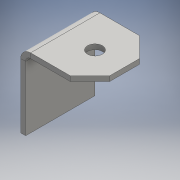
# Autodesk Inventor part: Part120
Saved by Autodesk Inventor 2016 (Build 200138000, 138)
## iProperties
Created: 2018-11-16
Part Number: Part120
Material: Generic
Document SubType Name: Sheet Metal
Designer: hovm
Density: 1 g/cm^3
Sheet Metal Rule: Default_mm
Appearance: Default
Author: hovm
Autodesk Inventor part; units mm, degrees
ref_plane "YZ Plane" through (0, 0, 0) normal (1, 0, 0) x (0, 1, 0)
ref_plane "XZ Plane" through (0, 0, 0) normal (0, 1, 0) x (-1, 0, 0)
ref_plane "XY Plane" through (0, 0, 0) normal (0, 0, 1) x (1, 0, 0)
sketch "Sketch1" plane through (0, 0, 0) normal (0, 0, 1) x (1, 0, 0)
  line L0 (-7, -7) -> (7, -7)
  line L1 (7, -7) -> (7, 7)
  line L2 (7, 7) -> (-7, 7)
  line L3 (-7, 7) -> (-7, -7)
  line L4 (-7, -7) -> (7, 7) construction
  line L5 (7, -7) -> (-7, 7) construction
  point P0 (0, 0)
  dimension "d0" = 14
  dimension "d1" = 14
  measures "d0" distance of L1.end L2.end
  measures "d1" distance of L0.end L1.end
extrude "Plate1" add sketch "Sketch1" along normal blind 1
sketch "Sketch2" plane through (-6, 7, 1) normal (-1, 0, 0) x (0, -1, 0)
  line L0 (14, 0) -> (0, 0)
  line L1 (0, 0) -> (0, -15)
  line L2 (0, -15) -> (14, -15)
  line L3 (14, -15) -> (14, 0)
  constraints: 6 end point, 1 horizontal, 1 perpendicular, 1 vertical
edge flange "Flange1" height 15 angle 90 thickness 1 bend radius 1 thickness toward (-1, 0, 0) relief tear relief width 1 relief depth 0.5 edges at (-7, 0, 0) wall of the first edge with corners at (-6, -7, 1) (-6, 7, 1) (-6, 7, -14) (-6, -7, -14)
bend "Bend1"
corner "Corner1"
sketch "Sketch3" plane through (0, 0, 1) normal (0, 0, 1) x (1, 0, 0)
  line L0 (7, -7) -> (7, 7) projected
  point P0 (0, 0)
  point P1 (1, 0)
  point P2 (7, 0)
  dimension "d13" = 6
  constraints: 1 horizontal alignment, 1 midpoint
  measures "d13" distance from line of L0 point (1, 0)
hole "Hole1" at (1, 0, 1) direction (0, 0, -1) diameter 3 depth 1 tip angle 118
chamfer "Corner Chamfer1" distance 4 angle 45 2 edges at (7, 7, 0.5) (7, -7, 0.5)
equation "\"d1\" = d0"
equation "\"d19\" = Thickness"
equation "\"d3\" = BendReliefWidth"
equation "\"d4\" = BendReliefDepth"
equation "\"d5\" = MinimumRemnant"
equation "\"d6\" = BendRadius"
equation "\"d9\" = BendRadius"
equation "\"d10\" = CornerReliefSize"
equation "\"d11\" = GapSize"
equation "\"d12\" = JacobiRadiusSize"
equation "\"BendRadius\" = Thickness"
equation "\"BendReliefWidth\" = Thickness"
equation "\"BendReliefDepth\" = 0.5 * Thickness"
equation "\"CornerReliefSize\" = 4 * Thickness"
equation "\"MinimumRemnant\" = 2 * Thickness"
equation "\"TransitionRadius\" = BendRadius"
equation "\"JacobiRadiusSize\" = BendRadius"
equation "\"GapSize\" = Thickness"
equation "\"d2\" = BendRadius"
equation "\"Thickness\" = 1"
body "Solid1"
